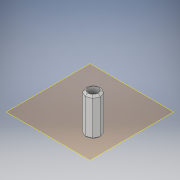
# Autodesk Inventor part: pin_oct_4mm
Saved by Autodesk Inventor 2019 (Build 230136000, 136)
## iProperties
Created: 2018-12-20
Part Number: pin_oct_4mm
Material: Generic
Document SubType Name: Modeling
Designer: assman
Density: 1 g/cm^3
Appearance: Default
Author: assman
## iProperties of the stored document pin_oct_4mm_3DPrint.ipt
Created: 2018-12-20
Part Number: pin_oct_4mm_3DPrint
Material: Generic
Document SubType Name: Modeling
Designer: assman
Density: 1 g/cm^3
Appearance: Default
Author: assman
Autodesk Inventor part; units mm, degrees
ref_plane "YZ Plane" through (0, 0, 0) normal (1, 0, 0) x (0, 1, 0)
ref_plane "XZ Plane" through (0, 0, 0) normal (0, 1, 0) x (-1, 0, 0)
ref_plane "XY Plane" through (0, 0, 0) normal (0, 0, 1) x (1, 0, 0)
ref_plane "Work Plane1" through (-10, 7, -20) normal (0, 1, 0) x (1, 0, 0)
sketch "Sketch3" plane through (-10, 7, -20) normal (0, 1, 0) x (1, 0, 0)
  circle A0 centre (5.4301, -4.6077) radius 2 construction
  line L0 (4.1095, -3.1058) -> (5.5583, -2.6118)
  line L1 (5.5583, -2.6118) -> (6.9321, -3.287)
  line L2 (6.9321, -3.287) -> (7.426, -4.7359)
  line L3 (7.426, -4.7359) -> (6.7508, -6.1096)
  line L4 (6.7508, -6.1096) -> (5.302, -6.6036)
  line L5 (5.302, -6.6036) -> (3.9282, -5.9284)
  line L6 (3.9282, -5.9284) -> (3.4343, -4.4795)
  line L7 (3.4343, -4.4795) -> (4.1095, -3.1058)
  point P0 (10, -20)
  constraints: 16 end point, 1 coincident, 19 other
extrude "Extrusion1" add sketch "Sketch3" along normal blind 10
chamfer "Chamfer1" distance 0.5 angle 45 8 edges at (-3.9736, 7, -13.6434) (-2.9116, 7, -14.5772) (-2.8209, 7, -15.9886) (-3.7548, 7, -17.0506) (-5.1661, 7, -17.1412) (-6.2281, 7, -16.2073) (-6.3188, 7, -14.796) (-5.3849, 7, -13.734)
chamfer "Chamfer2" distance 0.5 angle 45 8 edges at (-5.3849, 17, -13.734) (-3.9736, 17, -13.6434) (-6.3188, 17, -14.796) (-6.2281, 17, -16.2073) (-5.1661, 17, -17.1412) (-3.7548, 17, -17.0506) (-2.8209, 17, -15.9886) (-2.9116, 17, -14.5772)
sketch "Sketch4" plane through (-10, 17, -20) normal (0, 1, 0) x (1, 0, 0)
  line L0 (5.5236, -3.1519) -> (6.5257, -3.6444) construction
  line L1 (4.4668, -3.5122) -> (5.5236, -3.1519) construction
  line L2 (3.9743, -4.5142) -> (4.4668, -3.5122) construction
  line L3 (4.3346, -5.571) -> (3.9743, -4.5142) construction
  line L4 (5.3367, -6.0635) -> (4.3346, -5.571) construction
  line L5 (6.3935, -5.7032) -> (5.3367, -6.0635) construction
  line L6 (6.886, -4.7012) -> (6.3935, -5.7032) construction
  line L7 (6.5257, -3.6444) -> (6.886, -4.7012) construction
  point P0 (10, -20)
  point P1 (5.4301, -4.6077)
hole "Hole1" at (-4.5699, 17, -15.3923) direction (0, -1, 0) diameter 2.5 end through all
body "Solid2"
body "Solid1"
